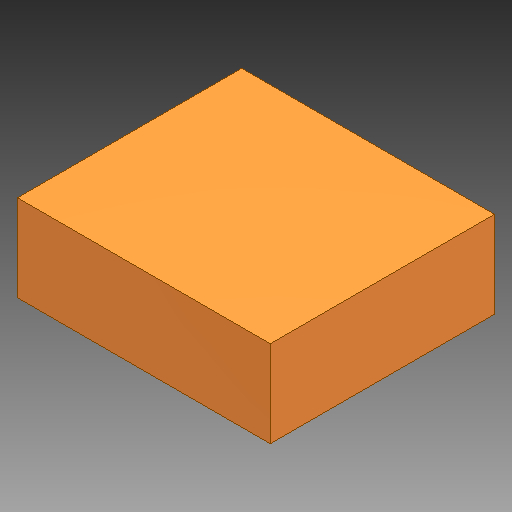
# Autodesk Inventor part: 2N7002
Saved by Autodesk Inventor 2017.3 (Build 213256000, 256)
## iProperties
Part Number: 2N7002
Material: Generisch
Document SubType Name: Modeling
Designer: Nils
Density: 1 g/cm^3
Appearance: SOT23, 2N7002
Author: Nils
Autodesk Inventor part; units mm, degrees
ref_plane "YZ Plane" through (0, 0, 0) normal (1, 0, 0) x (0, 1, 0)
ref_plane "XZ Plane" through (0, 0, 0) normal (0, 1, 0) x (-1, 0, 0)
ref_plane "XY Plane" through (0, 0, 0) normal (0, 0, 1) x (1, 0, 0)
sketch "SOT23, 2N7002_26" plane through (0, 0, 0) normal (0, 0, 1) x (1, 0, 0)
  line L0 (-1.4224, 1.2954) -> (1.4986, 1.2954)
  line L1 (1.4986, 1.2954) -> (1.4986, -1.2954)
  line L2 (1.4986, -1.2954) -> (-1.4224, -1.2954)
  line L3 (-1.4224, -1.2954) -> (-1.4224, 1.2954)
  constraints: 8 end point
extrude "Extrusion1" add sketch "SOT23, 2N7002_26" along normal blind 1
